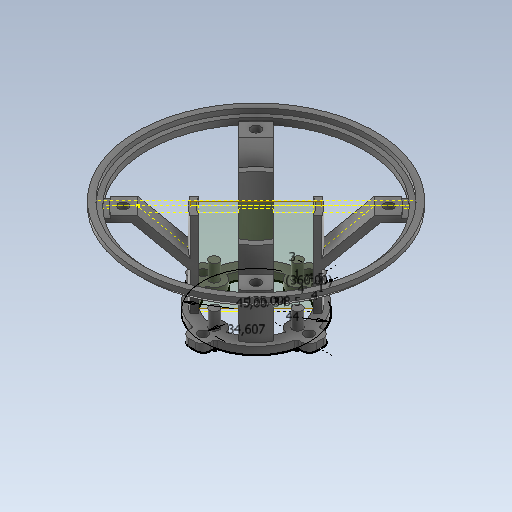
# Autodesk Inventor part: upper_mount001_beta
Saved by Autodesk Inventor 2020 (Build 240168000, 168)
## iProperties
Created: 2024-01-17
Part Number: upper_mount001_beta
Material: Типовые
Document SubType Name: Modeling
Designer: 4s
Density: 1 g/cm^3
Appearance: Гладкая — черная
Author: 4s
Autodesk Inventor part; units mm, degrees
sketch "Эскиз1" plane through (0, 0, 0) normal (0, 1, 0) x (-1, 0, 0)
  arc A0 (5.2609, -21.3617) -> (21.3617, -5.2609) centre (0, 0) ccw
  circle A1 centre (0, -22) radius 2
  line L0 (0, 0) -> (0, -33.2947) construction
  line L1 (0, 0) -> (-32.7614, 0) construction
  circle A2 centre (-22, 0) radius 2
  circle A3 centre (0, 22) radius 2
  circle A4 centre (22, 0) radius 2
  line L2 (4.5, -22) -> (-4.5, -22) construction
  line L3 (0, -22) -> (0, -26.5) construction
  line L4 (4.5, -22.3327) -> (4.5, -23.5)
  line L5 (1.5, -26.5) -> (-1.5, -26.5)
  line L6 (-4.5, -22.3327) -> (-4.5, -23.5)
  arc A5 (1.5, -26.5) -> (4.5, -23.5) centre (1.5, -23.5) ccw
  arc A6 (-4.5, -23.5) -> (-1.5, -26.5) centre (-1.5, -23.5) ccw
  arc A7 (1.9979, -21.9091) -> (4.5, -21.5349) centre (0, 0) ccw construction
  arc A8 (-4.5, -21.5349) -> (1.9979, -21.9091) centre (0, 0) ccw construction
  arc A9 (5.2609, -21.3617) -> (4.5, -22.3327) centre (5.5, -22.3327) ccw
  arc A10 (-4.5, -22.3327) -> (-5.2609, -21.3617) centre (-5.5, -22.3327) ccw
  line L7 (0, 0) -> (15.5563, -15.5563) construction
  line L8 (0, 0) -> (22, 0) construction
  line L9 (22.3327, -4.5) -> (23.5, -4.5)
  line L10 (26.5, -1.5) -> (26.5, 1.5)
  line L11 (22.3327, 4.5) -> (23.5, 4.5)
  arc A11 (23.5, -4.5) -> (26.5, -1.5) centre (23.5, -1.5) ccw
  arc A12 (26.5, 1.5) -> (23.5, 4.5) centre (23.5, 1.5) ccw
  arc A13 (22.3327, -4.5) -> (21.3617, -5.2609) centre (22.3327, -5.5) ccw
  arc A14 (21.3617, 5.2609) -> (22.3327, 4.5) centre (22.3327, 5.5) ccw
  line L12 (0, 0) -> (-15.5563, -15.5563) construction
  line L13 (0, 0) -> (22, 0) construction
  line L14 (-22.3327, 4.5) -> (-23.5, 4.5)
  line L15 (-26.5, 1.5) -> (-26.5, -1.5)
  line L16 (-22.3327, -4.5) -> (-23.5, -4.5)
  arc A15 (-23.5, 4.5) -> (-26.5, 1.5) centre (-23.5, 1.5) ccw
  arc A16 (-26.5, -1.5) -> (-23.5, -4.5) centre (-23.5, -1.5) ccw
  arc A17 (-22.3327, 4.5) -> (-21.3617, 5.2609) centre (-22.3327, 5.5) ccw
  arc A18 (-21.3617, -5.2609) -> (-22.3327, -4.5) centre (-22.3327, -5.5) ccw
  arc A19 (-5.2609, 21.3617) -> (-4.5, 22.3327) centre (-5.5, 22.3327) ccw
  line L17 (-4.5, 22.3327) -> (-4.5, 23.5)
  arc A20 (-1.5, 26.5) -> (-4.5, 23.5) centre (-1.5, 23.5) ccw
  line L18 (-1.5, 26.5) -> (1.5, 26.5)
  arc A21 (4.5, 23.5) -> (1.5, 26.5) centre (1.5, 23.5) ccw
  line L19 (4.5, 22.3327) -> (4.5, 23.5)
  arc A22 (4.5, 22.3327) -> (5.2609, 21.3617) centre (5.5, 22.3327) ccw
  arc A23 (21.3617, -5.2609) -> (21.3617, 5.2609) centre (0, 0) ccw construction
  arc A24 (21.3617, 5.2609) -> (5.2609, 21.3617) centre (0, 0) ccw
  arc A25 (5.2609, 21.3617) -> (-5.2609, 21.3617) centre (0, 0) ccw construction
  arc A26 (-5.2609, 21.3617) -> (-21.3617, 5.2609) centre (0, 0) ccw
  arc A27 (-21.3617, 5.2609) -> (-21.3617, -5.2609) centre (0, 0) ccw construction
  arc A28 (-21.3617, -5.2609) -> (-5.2609, -21.3617) centre (0, 0) ccw
  circle A29 centre (0, 0) radius 17
  circle A30 centre (0, -17.3035) radius 2
  circle A31 centre (0, 17.3035) radius 2
  circle A32 centre (-17.3035, 0) radius 2
  circle A33 centre (17.3035, 0) radius 2
  arc A34 (4.1696, -16.4807) -> (-4.1696, -16.4807) centre (0, -17.3035) ccw
  arc A35 (-16.4807, -4.1696) -> (-16.4807, 4.1696) centre (-17.3035, 0) ccw
  arc A36 (16.4807, 4.1696) -> (16.4807, -4.1696) centre (17.3035, 0) ccw
  arc A37 (-4.1696, 16.4807) -> (4.1696, 16.4807) centre (0, 17.3035) ccw
  arc A38 (1.8099, -21.1489) -> (4.1696, -16.4807) centre (0, -17.3035) ccw construction
  arc A39 (-4.1696, -16.4807) -> (1.8099, -21.1489) centre (0, -17.3035) ccw construction
  arc A40 (-21.1489, -1.8099) -> (-16.4807, -4.1696) centre (-17.3035, 0) ccw construction
  arc A41 (-16.4807, 4.1696) -> (-21.1489, -1.8099) centre (-17.3035, 0) ccw construction
  arc A42 (-1.8099, 21.1489) -> (-4.1696, 16.4807) centre (0, 17.3035) ccw construction
  arc A43 (4.1696, 16.4807) -> (-1.8099, 21.1489) centre (0, 17.3035) ccw construction
  arc A44 (21.1489, 1.8099) -> (16.4807, 4.1696) centre (17.3035, 0) ccw construction
  arc A45 (16.4807, -4.1696) -> (21.1489, 1.8099) centre (17.3035, 0) ccw construction
  point P0 (4.5, -26.5)
  point P1 (-4.5, -26.5)
  point P2 (4.5, -26.5)
  point P3 (-4.5, -26.5)
  point P4 (-16.8871, 1.9562)
  point P5 (-16.8871, -1.9562)
  point P6 (-1.9562, -16.8871)
  point P7 (1.9562, -16.8871)
  point P8 (16.8871, -1.9562)
  point P9 (16.8871, 1.9562)
  point P10 (1.9562, 16.8871)
  point P11 (-1.9562, 16.8871)
  dimension "d13" = 34
  dimension "d0" = 44
  dimension "d1" = 4
  dimension "d4" = 360
  dimension "d6" = 9
  dimension "d7" = 4.5
  dimension "d8" = 3
  dimension "d9" = 1
  dimension "d10" = 1
  dimension "d11" = 45
  dimension "d12" = 135
  dimension "d73" = 4
  dimension "d74" = 34.607
  dimension "d75" = 8.5
  constraints: 84 point on circle, 44 symmetric about line, 42 centre point, 40 end point, 12 point on line, 8 tangent, 6 coincident, 5 horizontal, 3 midpoint, 3 vertical, 2 equal length, 1 equal radius, 46 other
  measures "d0" diameter of A0
  measures "d1" diameter of A1
  measures "d6" distance of L2.start L2.end
  measures "d7" distance of L3.start L3.end
  measures "d8" radius of A5
  measures "d9" radius of A9
  measures "d10" radius of A10
  measures "d11" angle of L7 L8
  measures "d12" angle of L12 L13
  measures "d73" diameter of A30
  measures "d74" distance of A31.centre A30.centre
  measures "d75" diameter of A34
extrude "Выдавливание1" add sketch "Эскиз1" along normal blind 3 contours A9 L4 A5 L5 A6 L6 A10 A28 A18 L16 A16 L15 A15 L14 A17 A26 A19 L17 A20 L18 A21 L19 A22 A24 A14 L11 A12 L10 A11 L9 A13 A0 | A33 A29 | A29 A31 | A30 A29 | A29 A32 picked at (17.6987, -0.5048) picked at (-0.0698, 17.7558) picked at (-0.0698, -17.7558) picked at (-17.7548, 0.0789)
sketch "Эскиз2" plane through (0, 3, 0) normal (0, 1, 0) x (1, 0, 0)
  circle A0 centre (0, 0) radius 17 projected
  arc A1 (20, 0) -> (-17.2286, -10.1575) centre (0, 0) ccw construction
  line L0 (0, 0) -> (-14.1421, 14.1421) construction
  line L1 (0, 0) -> (20, 0) construction
  line L2 (0, 0) -> (-14.1421, -14.1421) construction
  line L3 (0, 0) -> (-20, 0) construction
  line L4 (0, 0) -> (0, 20) construction
  line L5 (-10.1575, -17.2286) -> (-7.9536, -15.0247)
  line L6 (-17.2286, -10.1575) -> (-15.0247, -7.9536)
  arc A2 (-10.1575, -17.2286) -> (20, 0) centre (0, 0) ccw construction
  arc A3 (-17.2286, -10.1575) -> (-10.1575, -17.2286) centre (0, 0) ccw
  line L7 (-10.1575, 17.2286) -> (-7.9536, 15.0247)
  line L8 (-17.2286, 10.1575) -> (-15.0247, 7.9536)
  arc A4 (-10.1575, 17.2286) -> (-17.2286, 10.1575) centre (0, 0) ccw
  line L9 (10.1575, -17.2286) -> (7.9536, -15.0247)
  line L10 (17.2286, -10.1575) -> (15.0247, -7.9536)
  arc A5 (10.1575, -17.2286) -> (17.2286, -10.1575) centre (0, 0) ccw
  line L11 (17.2286, 10.1575) -> (15.0247, 7.9536)
  arc A6 (17.2286, 10.1575) -> (10.1575, 17.2286) centre (0, 0) ccw
  line L12 (10.1575, 17.2286) -> (7.9536, 15.0247)
  circle A7 centre (0, 0) radius 17.5
  point P0 (15.0247, -7.9536)
  point P1 (7.9536, -15.0247)
  point P2 (7.9536, 15.0247)
  point P3 (15.0247, 7.9536)
  point P4 (-15.0247, 7.9536)
  point P5 (-7.9536, 15.0247)
  point P6 (-15.0247, -7.9536)
  point P7 (-8.323, -15.3941)
  point P8 (-15.3941, -8.323)
  point P9 (-15.3941, 8.323)
  point P10 (-8.323, 15.3941)
  point P11 (8.323, 15.3941)
  point P12 (15.3941, 8.323)
  point P13 (15.3941, -8.323)
  point P14 (8.323, -15.3941)
  dimension "d16" = 3
  dimension "d17" = 135
  dimension "d19" = 5
  dimension "d71" = 35
  constraints: 26 end point, 20 point on circle, 14 symmetric about line, 7 centre point, 2 coincident, 2 horizontal, 1 equal length, 1 parallel, 1 vertical, 6 other
  measures "d17" angle of L1 L0
  measures "d19" distance between parallel lines of L2 L5
  measures "d71" diameter of A7
extrude "Выдавливание2" add sketch "Эскиз2" along normal blind 35 contours A7 L12 A6 L11 | L10 A5 L9 A7 | A7 L8 A4 L7 | L5 A3 L6 A7
sketch "Эскиз3" plane through (0, 38, 0) normal (0, 1, 0) x (1, 0, 0)
  circle A0 centre (0, 0) radius 46
  circle A1 centre (0, 0) radius 16
  dimension "d22" = 92
  dimension "d23" = 32
  constraints: 2 centre point, 1 coincident
  measures "d22" diameter of A0
  measures "d23" diameter of A1
sketch "Эскиз4" plane through (15.0247, 3, 7.9536) normal (0.7071068, 0, -0.7071068) x (-0.7071068, 0, -0.7071068)
  line L0 (62.2481, 35) -> (-29.7519, 35) construction
  line L1 (-3.1168, 0) -> (-3.1168, 35) construction
  line L2 (-22.7519, 35) -> (-3.1168, 15.3649)
  line L3 (-18.5093, 35) -> (-3.1168, 19.6076)
  line L4 (-3.1168, 15.3649) -> (-3.1168, 19.6076)
  line L5 (-22.7519, 35) -> (-18.5093, 35)
  line L6 (-3.1168, 0) -> (-3.1168, 0) projected
  line L7 (-3.1168, 0) -> (-3.1168, 35) projected
  line L8 (-3.1168, 0) -> (-3.1168, 35) projected
  line L9 (-3.1168, 35) -> (-3.1168, 35) projected
  point P0 (16.2481, -3)
  dimension "d26" = 45
  dimension "d27" = 7
  dimension "d28" = 3
  constraints: 8 end point, 4 point on line, 2 collinear, 1 parallel
  measures "d26" angle of L0 L2
  measures "d27" distance of L0.end L2.start
  measures "d28" distance between parallel lines of L2 L3
extrude "Выдавливание4" add sketch "Эскиз4" against normal blind 10
pattern_circular "Круговой массив1" count 4 over 360 about axis through (0, -10, 0) along (0, 1, 0) of "Выдавливание4", "Выдавливание2"
ref_plane "РабПлоскость2" through (0, 39, 0) normal (0, 1, 0) x (1, 0, 0)
sketch "Эскиз5" plane through (0, 39, 0) normal (0, 1, 0) x (1, 0, 0)
  arc A0 (10.1575, -17.2286) -> (17.2286, -10.1575) centre (0, 0) ccw construction
  arc A1 (-17.2286, -10.1575) -> (-10.1575, -17.2286) centre (0, 0) ccw construction
  arc A2 (-15.0247, -7.9536) -> (-7.9536, -15.0247) centre (0, 0) ccw construction
  arc A3 (-7.9536, 15.0247) -> (-15.0247, 7.9536) centre (0, 0) ccw construction
  arc A4 (-10.1575, 17.2286) -> (-17.2286, 10.1575) centre (0, 0) ccw construction
  arc A5 (17.2286, 10.1575) -> (10.1575, 17.2286) centre (0, 0) ccw construction
  circle A6 centre (0, 0) radius 17 construction
  circle A7 centre (0, 0) radius 17 projected
  arc A8 (17.2286, 10.1575) -> (10.1575, 17.2286) centre (0, 0) ccw construction
  arc A9 (-10.1575, 17.2286) -> (-17.2286, 10.1575) centre (0, 0) ccw construction
  arc A10 (-17.2286, -10.1575) -> (-10.1575, -17.2286) centre (0, 0) ccw construction
  arc A11 (10.1575, -17.2286) -> (17.2286, -10.1575) centre (0, 0) ccw construction
  line L0 (17.2286, -10.1575) -> (28.1127, -21.0416) construction
  line L1 (31.1127, -24.0416) -> (17.2286, -10.1575) construction
  line L2 (15.3941, -8.323) -> (17.2286, -10.1575) construction
  line L3 (17.2286, 10.1575) -> (15.3941, 8.323) construction
  line L4 (17.2286, 10.1575) -> (31.1127, 24.0416) construction
  line L5 (28.1127, 21.0416) -> (17.2286, 10.1575) construction
  line L6 (-8.323, -15.3941) -> (-10.1575, -17.2286) construction
  line L7 (-10.1575, -17.2286) -> (-21.0416, -28.1127) construction
  line L8 (-24.0416, -31.1127) -> (-10.1575, -17.2286) construction
  line L9 (10.1575, -17.2286) -> (24.0416, -31.1127) construction
  line L10 (21.0416, -28.1127) -> (10.1575, -17.2286) construction
  line L11 (10.1575, -17.2286) -> (8.323, -15.3941) construction
  arc A12 (17.2286, 10.1575) -> (10.1575, 17.2286) centre (0, 0) ccw construction
  line L12 (-17.2286, -10.1575) -> (-15.3941, -8.323) construction
  line L13 (-17.2286, -10.1575) -> (-31.1127, -24.0416) construction
  line L14 (-28.1127, -21.0416) -> (-17.2286, -10.1575) construction
  line L15 (8.323, 15.3941) -> (10.1575, 17.2286) construction
  line L16 (10.1575, 17.2286) -> (21.0416, 28.1127) construction
  line L17 (24.0416, 31.1127) -> (10.1575, 17.2286) construction
  line L18 (-10.1575, 17.2286) -> (-8.323, 15.3941) construction
  line L19 (-10.1575, 17.2286) -> (-24.0416, 31.1127) construction
  line L20 (-21.0416, 28.1127) -> (-10.1575, 17.2286) construction
  line L21 (-15.3941, 8.323) -> (-17.2286, 10.1575) construction
  line L22 (-17.2286, 10.1575) -> (-28.1127, 21.0416) construction
  line L23 (-31.1127, 24.0416) -> (-17.2286, 10.1575) construction
  circle A13 centre (0, 0) radius 17 construction
  circle A14 centre (0, 0) radius 20
  circle A15 centre (0, 0) radius 7.75
  line L24 (-17.2286, 10.1575) -> (-15.3941, 8.323) projected
  line L25 (-28.1127, 21.0416) -> (-31.1127, 24.0416) projected
  line L26 (-8.323, 15.3941) -> (-10.1575, 17.2286) projected
  line L27 (-24.0416, 31.1127) -> (-21.0416, 28.1127) projected
  line L28 (10.1575, 17.2286) -> (8.323, 15.3941) projected
  line L29 (21.0416, 28.1127) -> (24.0416, 31.1127) projected
  line L30 (-15.3941, -8.323) -> (-17.2286, -10.1575) projected
  line L31 (-31.1127, -24.0416) -> (-28.1127, -21.0416) projected
  line L32 (24.0416, -31.1127) -> (21.0416, -28.1127) projected
  line L33 (8.323, -15.3941) -> (10.1575, -17.2286) projected
  line L34 (-10.1575, -17.2286) -> (-8.323, -15.3941) projected
  line L35 (-21.0416, -28.1127) -> (-24.0416, -31.1127) projected
  line L36 (15.3941, 8.323) -> (17.2286, 10.1575) projected
  line L37 (31.1127, 24.0416) -> (28.1127, 21.0416) projected
  line L38 (28.1127, -21.0416) -> (31.1127, -24.0416) projected
  line L39 (17.2286, -10.1575) -> (15.3941, -8.323) projected
  arc A16 (10.1575, -17.2286) -> (17.2286, -10.1575) centre (0, 0) ccw projected
  arc A17 (10.1575, -17.2286) -> (17.2286, -10.1575) centre (0, 0) ccw projected
  arc A18 (10.1575, -17.2286) -> (17.2286, -10.1575) centre (0, 0) ccw projected
  arc A19 (-17.2286, -10.1575) -> (-10.1575, -17.2286) centre (0, 0) ccw projected
  arc A20 (-17.2286, -10.1575) -> (-10.1575, -17.2286) centre (0, 0) ccw projected
  arc A21 (-17.2286, -10.1575) -> (-10.1575, -17.2286) centre (0, 0) ccw projected
  arc A22 (-10.1575, 17.2286) -> (-17.2286, 10.1575) centre (0, 0) ccw projected
  arc A23 (-10.1575, 17.2286) -> (-17.2286, 10.1575) centre (0, 0) ccw projected
  arc A24 (-10.1575, 17.2286) -> (-17.2286, 10.1575) centre (0, 0) ccw projected
  arc A25 (17.2286, 10.1575) -> (10.1575, 17.2286) centre (0, 0) ccw projected
  arc A26 (17.2286, 10.1575) -> (10.1575, 17.2286) centre (0, 0) ccw projected
  arc A27 (17.2286, 10.1575) -> (10.1575, 17.2286) centre (0, 0) ccw projected
  dimension "d36" = 15.5
  constraints: 3 centre point, 3 coincident, 1 concentric, 1 other
  measures "d36" diameter of A15
ref_plane "РабПлоскость1" through (0, 39, 0) normal (0, 1, 0) x (1, 0, 0)
sketch "Эскиз6" plane through (0, 39, 0) normal (0, 1, 0) x (1, 0, 0)
  point P0 (0, 0)
sketch "Эскиз7" plane through (-24.0416, 38, 31.1127) normal (0, 1, 0) x (0.7071068, 0, 0.7071068)
  circle A0 centre (-5, 39) radius 44 construction
  circle A1 centre (-5, 39) radius 46 construction
  line L0 (-39.7574, 34) -> (-44, 34) construction
  line L1 (-39.7574, 34) -> (-39.7574, 44) construction
  line L2 (-44, 44) -> (-39.7574, 44) construction
  line L3 (-44, 34) -> (-44, 44) construction
  line L4 (-10, 73.7574) -> (-10, 78) construction
  line L5 (-10, 73.7574) -> (0, 73.7574) construction
  line L6 (0, 78) -> (0, 73.7574) construction
  line L7 (-10, 78) -> (0, 78) construction
  line L8 (29.7574, 44) -> (34, 44) construction
  line L9 (29.7574, 44) -> (29.7574, 34) construction
  line L10 (34, 34) -> (29.7574, 34) construction
  line L11 (34, 44) -> (34, 34) construction
  line L12 (0, 4.2426) -> (0, 0) construction
  line L13 (0, 4.2426) -> (-10, 4.2426) construction
  line L14 (-10, 0) -> (-10, 4.2426) construction
  line L15 (0, 0) -> (-10, 0) construction
  line L16 (-10, 78) -> (0, 78) construction
  line L17 (-5, 85) -> (-5, -5) construction
  line L18 (0, 0) -> (-10, 0) construction
  line L19 (-44, 34) -> (-44, 44) construction
  line L20 (-49, 39) -> (39, 39) construction
  circle A2 centre (-5, 83) radius 0.35 construction
  circle A3 centre (-5, 39) radius 7.75 construction
  circle A4 centre (-6.27, 82.9817) radius 0.35 construction
  circle A5 centre (-3.73, 82.9817) radius 0.35 construction
  line L21 (-5, 39) -> (-5, 78) construction
  circle A6 centre (-5, 39) radius 47
  circle A7 centre (-5, 39) radius 49.5
  line L22 (-10, 73.7574) -> (-10, 85.7333)
  line L23 (-10, 78) -> (-10, 58.3649) projected
  line L24 (-10, 73.7574) -> (0, 73.7574) projected
  line L25 (-10, 73.7574) -> (0, 73.7574)
  line L26 (0, 73.7574) -> (0, 85.7333)
  line L27 (-5, 39) -> (9.0563, 53.0563) construction
  line L28 (29.7574, 34) -> (41.7333, 34)
  line L29 (29.7574, 34) -> (29.7574, 44)
  line L30 (29.7574, 44) -> (41.7333, 44)
  line L31 (9.0563, 24.9437) -> (-19.1449, 53.1449) construction
  line L32 (-39.7574, 44) -> (-51.7333, 44)
  line L33 (-39.7574, 44) -> (-39.7574, 34)
  line L34 (-39.7574, 34) -> (-51.7333, 34)
  line L35 (-10, 4.2426) -> (-10, -7.7333)
  line L36 (0, 4.2426) -> (-10, 4.2426)
  line L37 (0, 4.2426) -> (0, -7.7333)
  point P0 (-5, 39)
  point P1 (-5, 83.35)
  point P2 (41.7333, 34)
  point P3 (41.7333, 44)
  point P4 (-10, -7.7333)
  point P5 (0, -7.7333)
  dimension "d4" = 360
  dimension "d40" = 0.7
  dimension "d37" = 88
  dimension "d45" = 0.7
  dimension "d46" = 1.27
  dimension "d47" = 0.7
  dimension "d48" = 1.27
  dimension "d49" = 0
  dimension "d50" = 2
  dimension "d51" = 1
  dimension "d52" = 2.5
  constraints: 34 end point, 8 point on circle, 6 symmetric about line, 5 centre point, 4 coincident, 3 midpoint, 3 point on line, 2 collinear, 2 vertical alignment, 1 perpendicular, 4 other
  measures "d37" diameter of A0
  measures "d45" diameter of A4
  measures "d46" horizontal distance of point (-5, 83) A4.centre
  measures "d47" diameter of A5
  measures "d48" horizontal distance of A5.centre point (-5, 83)
  measures "d49" distance between parallel lines of L21 L17
  measures "d52" radial gap between concentric circles of A6 A7
extrude "Выдавливание6" add sketch "Эскиз7" along normal blind 2
sketch "Эскиз8" plane through (0, 39, 0) normal (0, 1, 0) x (1, 0, 0)
  point P0 (0, 0)
extrude "Выдавливание7" add sketch "Эскиз7" against normal blind 2.5 contours A6 L28 L29 L30 | L26 L24 L22 A6 | A6 L35 L36 L37 | L32 L33 L34 A6
sketch "Эскиз9" plane through (0, 0, 0) normal (1, 0, 0) x (0, 1, 0)
  point P0 (0, 0)
ref_plane "РабПлоскость3" through (-31.1127, 38, -31.1127) normal (-0.7071068, 0, 0.7071068) x (0.7071068, 0, 0.7071068)
sketch "Эскиз10" plane through (-31.1127, 38, -31.1127) normal (-0.7071068, 0, 0.7071068) x (0.7071068, 0, 0.7071068)
  line L0 (90.7333, 0) -> (90.7333, 0) projected
  line L1 (90.7333, 0) -> (90.7333, -2.5) projected
  line L2 (90.7333, -2.5) -> (90.7333, -2.5) projected
  line L3 (90.7333, 0) -> (90.7333, -2.5) projected
  line L4 (93.5, 2) -> (-5.5, 2) projected
  line L5 (93.5, 0) -> (-5.5, 0) projected
  line L6 (93.5, 0) -> (-5.5, 0) projected
  line L7 (93.5, 0) -> (91, -2.5)
  line L8 (93.5, 0) -> (91, 0)
  line L9 (91, 0) -> (91, -2.5)
  line L10 (91, -2.5) -> (88, -2.5)
  line L11 (90.7333, -2.5) -> (80.5, -2.5) projected
  line L12 (88, -2.5) -> (88, 0)
  line L13 (49, 0) -> (90.7333, 0) projected
  line L14 (88, 0) -> (93.5, 0)
  point P0 (44, -38)
  dimension "d58" = 3
  constraints: 12 end point, 2 collinear, 2 point on line, 1 perpendicular
  measures "d58" distance of L9.end L10.end
sketch "Эскиз11" plane through (-31.1127, 38, -31.1127) normal (-0.7071068, 0, 0.7071068) x (0.7071068, 0, 0.7071068)
  line L0 (93.5, 2) -> (-5.5, 2) projected
  line L1 (93.5, 0) -> (-5.5, 0) projected
  line L2 (-2.7333, 0) -> (-2.7333, 0) projected
  line L3 (-2.7333, 0) -> (-2.7333, -2.5) projected
  line L4 (-2.7333, -2.5) -> (-2.7333, -2.5) projected
  line L5 (-2.7333, 0) -> (-2.7333, -2.5) projected
  line L6 (9.2426, 0) -> (-2.7333, 0) projected
  line L7 (-2.7333, 0) -> (-2.7333, -2.5) projected
  line L8 (7.5, -2.5) -> (-2.7333, -2.5) projected
  line L9 (7.5, -2.5) -> (24.6351, -19.6351) projected
  line L10 (24.6351, -35) -> (24.6351, -19.6351) projected
  line L11 (27.2295, -35) -> (24.6351, -35) projected
  line L12 (24.6351, 0) -> (27.2295, 0) projected
  line L13 (24.6351, -15.3924) -> (24.6351, 0) projected
  line L14 (24.6351, -15.3924) -> (9.2426, 0) projected
  line L15 (93.5, 0) -> (-5.5, 0) projected
  line L16 (-3, -2.5) -> (-2.7333, -2.5) projected
  line L17 (-5.5, 0) -> (-3, -2.5)
  line L18 (-3, -2.5) -> (-1, -2.5)
  line L19 (-2.7333, -2.5) -> (7.5, -2.5) projected
  line L20 (-1, -2.5) -> (-1, 0)
  line L21 (-2.7333, 0) -> (39, 0) projected
  line L22 (-5.5, 0) -> (-1, 0)
  line L23 (27.2295, -35) -> (27.2295, 0) projected
  point P0 (44, -38)
  point P1 (27.7519, 0)
  point P2 (-1, -2.5)
  point P3 (-1, 0)
  dimension "d59" = 2
  constraints: 8 end point, 2 point on line, 1 collinear, 1 perpendicular
  measures "d59" distance of L16.start L18.end
sketch3d "3D эскиз1"
  arc A0 (35.0018, 38, 35.0018) -> (35.0018, 38, -35.0018) centre (0, 38, 0) ccw
  arc A1 (35.0018, 38, -35.0018) -> (-35.0018, 38, -35.0018) centre (0, 38, 0) ccw
  arc A2 (-35.0018, 38, -35.0018) -> (-35.0018, 38, 35.0018) centre (0, 38, 0) ccw
  arc A3 (-35.0018, 38, 35.0018) -> (35.0018, 38, 35.0018) centre (0, 38, 0) ccw
sweep "Сдвиг1" add profiles "Эскиз11" path "3D эскиз1" contours L20 L8 L3 L1 | L3 L16 L17 L1
sketch "Эскиз12" plane through (0, 38, 0) normal (0, 1, 0) x (1, 0, 0)
  circle A0 centre (0, 0) radius 44 construction
  circle A1 centre (0, 0) radius 43
  circle A2 centre (0, 0) radius 45
  point P0 (0, 0)
  dimension "d62" = 1
  dimension "d63" = 1
  constraints: 2 centre point, 2 coincident
  measures "d62" radial gap between concentric circles of A0 A1
  measures "d63" radial gap between concentric circles of A0 A2
extrude "Выдавливание8" cut sketch "Эскиз12" against normal blind 1
sketch "Эскиз13" plane through (-21.0416, 38, 28.1127) normal (0, 1, 0) x (-0.7071068, 0, 0.7071068)
  circle A0 centre (-34.7574, -5) radius 17 projected
  circle A1 centre (-34.7574, -5) radius 39 construction
  line L0 (-34.7574, -5) -> (-34.7574, 34) construction
  line L1 (-34.7574, -5) -> (4.2426, -5) construction
  line L2 (-34.7574, -5) -> (-7.1802, 22.5772) construction
  line L3 (-34.7574, -5) -> (4.2426, -5) construction
  circle A2 centre (-34.7574, 34) radius 2
  circle A3 centre (4.2426, -5) radius 2
  line L4 (-34.7574, -5) -> (-62.3345, 22.5772) construction
  circle A4 centre (-73.7574, -5) radius 2
  circle A5 centre (-34.7574, -44) radius 2
  dimension "d66" = 78
  dimension "d67" = 45
  dimension "d68" = 4
  dimension "d72" = 45
  constraints: 10 end point, 5 centre point, 4 point on circle, 3 symmetric about line, 2 coincident, 1 equal length, 1 horizontal, 1 perpendicular, 1 vertical, 3 other
  measures "d66" diameter of A1
  measures "d67" angle of L3 L2
  measures "d68" diameter of A2
  measures "d72" angle of L0 L4
extrude "Выдавливание9" cut sketch "Эскиз13" against normal blind 10 contours A2 | A3 | A4 | A5
sketch "Эскиз14" plane through (0, 3, 0) normal (0, 1, 0) x (1, 0, 0)
  point P0 (0, 0)
ref_plane "РабПлоскость4" through (-12.3744, 38, 12.3744) normal (-0.7071068, 0, -0.7071068) x (0.7071068, 0, -0.7071068)
sketch "Эскиз15" plane through (-12.3744, 38, 12.3744) normal (-0.7071068, 0, -0.7071068) x (0.7071068, 0, -0.7071068)
  line L0 (-1.8649, 19.6351) -> (-19, 2.5) construction
  line L1 (-1.8649, 19.6351) -> (-1.8649, 19.6351) construction
  line L2 (-19, 2.5) -> (-1.8649, 19.6351) construction
  line L3 (-25.2083, 1) -> (-25.2083, 0) construction
  line L4 (-17.2574, 0) -> (-25.2083, 0) construction
  line L5 (-17.2574, 0) -> (-1.8649, 15.3924) construction
  line L6 (-1.8649, 15.3924) -> (-1.8649, 0) construction
  line L7 (0.7295, 0) -> (-1.8649, 0) construction
  line L8 (0.7295, 35) -> (0.7295, 0) construction
  line L9 (-1.8649, 35) -> (0.7295, 35) construction
  line L10 (-1.8649, 35) -> (-1.8649, 19.6351) construction
  line L11 (-1.8649, 19.6351) -> (-19, 2.5) construction
  line L12 (-27.2214, 2.5) -> (-19, 2.5) construction
  line L13 (-27.2214, 2.5) -> (-27.2214, 1) construction
  line L14 (-27.2214, 1) -> (-25.2083, 1) construction
  line L15 (-1.4736, 38) -> (-2.299, 38) construction
  line L16 (-1.325, 38) -> (-1.4736, 38) construction
  line L17 (-1.325, 38) -> (-1.325, 38) construction
  line L18 (-1.4736, 38) -> (-1.325, 38) construction
  line L19 (-2.299, 38) -> (-1.4736, 38) construction
  line L20 (-2.299, 38) -> (-2.299, 38) construction
  line L21 (-0.1777, 38) -> (-2.299, 38) construction
  line L22 (4.065, 38) -> (-0.1777, 38) construction
  line L23 (4.8904, 38) -> (4.065, 38) construction
  line L24 (6.115, 38) -> (4.8904, 38) construction
  line L25 (28.885, 38) -> (6.115, 38) construction
  line L26 (30.1096, 38) -> (28.885, 38) construction
  line L27 (30.935, 38) -> (30.1096, 38) construction
  line L28 (35.1777, 38) -> (30.935, 38) construction
  line L29 (37.299, 38) -> (35.1777, 38) construction
  line L30 (37.299, 38) -> (37.299, 38) construction
  line L31 (36.4736, 38) -> (37.299, 38) construction
  line L32 (36.325, 38) -> (36.4736, 38) construction
  line L33 (36.325, 38) -> (36.325, 38) construction
  line L34 (36.4736, 38) -> (36.325, 38) construction
  line L35 (37.299, 38) -> (36.4736, 38) construction
  line L36 (37.299, 38) -> (37.299, 38) construction
  line L37 (35.1777, 38) -> (37.299, 38) construction
  line L38 (30.935, 38) -> (35.1777, 38) construction
  line L39 (30.1096, 38) -> (30.935, 38) construction
  line L40 (28.885, 38) -> (30.1096, 38) construction
  line L41 (6.115, 38) -> (28.885, 38) construction
  line L42 (4.8904, 38) -> (6.115, 38) construction
  line L43 (4.065, 38) -> (4.8904, 38) construction
  line L44 (-0.1777, 38) -> (4.065, 38) construction
  line L45 (-2.299, 38) -> (-0.1777, 38) construction
  line L46 (-2.299, 38) -> (-2.299, 38) construction
  line L47 (35.0563, 38) -> (31.0563, 38) construction
  line L48 (35.0563, 38) -> (31.0563, 38) construction
  line L49 (3.9437, 38) -> (-0.0563, 38) construction
  line L50 (3.9437, 38) -> (-0.0563, 38) construction
  line L51 (34.5, 38) -> (0.5, 38) construction
  arc A0 (12.5, 15.3924) -> (22.5, 15.3924) centre (17.5, 34.7574) ccw construction
  line L52 (22.5, 0) -> (12.5, 0) construction
  line L53 (12.5, 0) -> (22.5, 0) construction
  line L54 (64.5, -2) -> (-29.5, -2) construction
  line L55 (22.5, 0) -> (62.2214, 0) construction
  line L56 (-27.5, 0) -> (62.5, 0) construction
  line L57 (22.5, 1) -> (12.5, 1) construction
  line L58 (12.5, 2.5) -> (12.5, 1) construction
  line L59 (-27.2214, 2.5) -> (12.5, 2.5) construction
  line L60 (-27.2214, 1) -> (-27.2214, 2.5) construction
  line L61 (-27.2214, 1) -> (-27.2214, 1) construction
  line L62 (-27.2214, 2.5) -> (-27.2214, 1) construction
  line L63 (12.5, 2.5) -> (-27.2214, 2.5) construction
  line L64 (12.5, 1) -> (12.5, 2.5) construction
  line L65 (12.5, 1) -> (22.5, 1) construction
  line L66 (22.5, 2.5) -> (22.5, 1) construction
  line L67 (62.2214, 2.5) -> (22.5, 2.5) construction
  line L68 (62.2214, 1) -> (62.2214, 2.5) construction
  line L69 (62.2214, 1) -> (62.2214, 1) construction
  line L70 (62.2214, 2.5) -> (62.2214, 1) construction
  line L71 (22.5, 2.5) -> (62.2214, 2.5) construction
  line L72 (22.5, 1) -> (22.5, 2.5) construction
  line L73 (60.2083, 1) -> (62.2214, 1) construction
  line L74 (62.2214, 1) -> (62.2214, 2.5) construction
  line L75 (54, 2.5) -> (62.2214, 2.5) construction
  line L76 (54, 2.5) -> (36.8649, 19.6351) construction
  line L77 (36.8649, 35) -> (36.8649, 19.6351) construction
  line L78 (34.2705, 35) -> (36.8649, 35) construction
  line L79 (34.2705, 35) -> (34.2705, 0) construction
  line L80 (36.8649, 0) -> (34.2705, 0) construction
  line L81 (36.8649, 15.3924) -> (36.8649, 0) construction
  line L82 (36.8649, 15.3924) -> (52.2574, 0) construction
  line L83 (52.2574, 0) -> (60.2083, 0) construction
  line L84 (60.2083, 0) -> (60.2083, 1) construction
  point P0 (17.5, 38)
  point P1 (-17.2574, 0)
extrude "Выдавливание10" add sketch "Эскиз1" along normal blind 10 contours A33 A29 | A29 A33 | A31 A29 | A29 A31 | A30 A29 | A29 A30 | A32 A29 | A29 A32
extrude "Выдавливание11" add sketch "Эскиз1" along normal blind 3 contours A29 A33 A36 | A37 A29 A31 | A29 A30 A34 | A35 A29 A32
